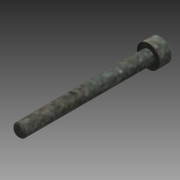
# Autodesk Inventor part: Screws
Saved by Autodesk Inventor 2016 (Build 200138000, 138)
## iProperties
Created: 2015-10-19
Part Number: Screws
Material: Steel
Document SubType Name: Modeling
Designer: Rus
Density: 7.85 g/cm^3
Appearance: Plate
Author: Rus
Autodesk Inventor part; units mm, degrees
ref_plane "YZ Plane" through (0, 0, 0) normal (1, 0, 0) x (0, 1, 0)
ref_plane "XZ Plane" through (0, 0, 0) normal (0, 1, 0) x (-1, 0, 0)
ref_plane "XY Plane" through (0, 0, 0) normal (0, 0, 1) x (1, 0, 0)
sketch "Sketch1" plane through (0, 0, 0) normal (0, 0, 1) x (1, 0, 0)
  line L0 (-2, -20) -> (-2, 20)
  line L1 (-2, 20) -> (2, 20)
  line L2 (2, 20) -> (2, -20)
  line L3 (2, -20) -> (-2, -20)
  line L4 (-2, -20) -> (2, 20) construction
  line L5 (-2, 20) -> (2, -20) construction
  line L6 (0, -20) -> (0, -19.6)
  line L7 (0, -20) -> (1.6, -20)
  line L8 (0, -20) -> (-1.6, -20)
  line L9 (-1.6, -20) -> (-2, -19.6)
  line L10 (0, 22.999163) -> (0, 17.000837)
  line L11 (0, 20) -> (0, 24)
  line L12 (0, 24) -> (3.5, 24)
  line L13 (0, 20) -> (3.5, 20)
  line L14 (3.5, 20) -> (3.5, 24)
  line L15 (0, 24) -> (-3.5, 24)
  line L16 (-3.5, 24) -> (-3.5, 20)
  line L17 (-3.5, 20) -> (0, 20)
  line L18 (0, 24) -> (3.1, 24)
  line L19 (0, 24) -> (0, 23.6)
  line L20 (3.1, 24) -> (3.5, 23.6)
  line L21 (0, 24) -> (-3.1, 24)
  line L22 (1.6, -20) -> (2, -19.6)
  line L23 (0, 20) -> (0, -20.824074)
  line L24 (0, -20) -> (0, 20)
  point P0 (0, 0)
  dimension "d0" = 40
  dimension "d1" = 4
  dimension "d2" = 0.4
  dimension "d3" = 1.6
  dimension "d4" = 1.6
  dimension "d5" = 4
  dimension "d6" = 3.5
  dimension "d7" = 3.5
  dimension "d8" = 3.1
  dimension "d9" = 0.4
  dimension "d10" = 3.1
  constraints: 50 end point, 12 point on line, 5 midpoint, 4 perpendicular, 3 vertical, 2 collinear, 2 parallel, 1 horizontal
  measures "d0" distance of L0.start L0.end
  measures "d1" distance of L0.end L1.end
  measures "d2" distance of L6.start L6.end
  measures "d3" distance of L6.start L7.end
  measures "d4" distance of L6.start L8.end
  measures "d5" distance of L11.start L11.end
  measures "d6" distance of L11.end L12.end
  measures "d7" distance of L11.end L15.end
  measures "d8" distance of L11.end L18.end
  measures "d9" distance of L11.end L19.end
  measures "d10" distance of L11.end L21.end
revolve "Revolution1" add sketch "Sketch1" angle 360 about axis through (0, -20, 0) along (0, 1, 0) contours L6 L23 L10 L1 L2 L22 L3 | L10 L11 L12 L20 L14 L13 L1
sketch "Sketch2" plane through (0, 24, 0) normal (0, 1, 0) x (1, 0, 0)
  line L0 (-2.8, -0.625) -> (2.8, -0.625)
  line L1 (2.8, -0.625) -> (2.8, 0.625)
  line L2 (2.8, 0.625) -> (-2.8, 0.625)
  line L3 (-2.8, 0.625) -> (-2.8, -0.625)
  line L4 (-2.8, -0.625) -> (2.8, 0.625) construction
  line L5 (2.8, -0.625) -> (-2.8, 0.625) construction
  line L6 (-0.625, -2.8) -> (-0.625, 2.8)
  line L7 (-0.625, 2.8) -> (0.625, 2.8)
  line L8 (0.625, 2.8) -> (0.625, -2.8)
  line L9 (0.625, -2.8) -> (-0.625, -2.8)
  circle A0 centre (0, 0) radius 2 projected
  line L10 (-0.625, -2.8) -> (0.625, 2.8) construction
  line L11 (-0.625, 2.8) -> (0.625, -2.8) construction
  dimension "d12" = 5.6
  dimension "d13" = 1.25
  dimension "d14" = 5.6
  dimension "d15" = 1.25
  constraints: 24 end point, 5 parallel, 4 midpoint, 2 perpendicular, 1 horizontal
  measures "d12" distance of L0.start L0.end
  measures "d13" distance of L1.end L0.end
  measures "d14" distance of L6.start L6.end
  measures "d15" distance of L6.end L7.end
sketch "Sketch2 outline for Extrusion1" plane through (0, 24, 0) normal (0, 1, 0) x (1, 0, 0)
  line L0 (-0.625, -2.8) -> (-0.625, -0.625)
  line L1 (0.625, -2.8) -> (-0.625, -2.8)
  line L2 (0.625, -0.625) -> (0.625, -2.8)
  line L3 (0.625, -0.625) -> (2.8, -0.625)
  line L4 (2.8, -0.625) -> (2.8, 0.625)
  line L5 (2.8, 0.625) -> (0.625, 0.625)
  line L6 (0.625, 2.8) -> (0.625, 0.625)
  line L7 (-0.625, 2.8) -> (0.625, 2.8)
  line L8 (-0.625, 0.625) -> (-0.625, 2.8)
  line L9 (-0.625, 0.625) -> (-2.8, 0.625)
  line L10 (-2.8, 0.625) -> (-2.8, -0.625)
  line L11 (-2.8, -0.625) -> (-0.625, -0.625)
extrude "Extrusion1" cut sketch "Sketch2 outline for Extrusion1" against normal blind 2.5 draft -10
body "Solid1"
